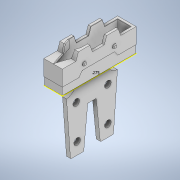
# Autodesk Inventor part: full bracket
Saved by Autodesk Inventor 2021 (Build 250183000, 183)
## iProperties
Created: 2021-07-17
Part Number: full bracket
Material: Generic
Document SubType Name: Modeling
Designer: newic
Density: 1 g/cm^3
Appearance: Default
Author: newic
Autodesk Inventor part; units mm, degrees
ref_plane "YZ Plane" through (0, 0, 0) normal (1, 0, 0) x (0, 1, 0)
ref_plane "XZ Plane" through (0, 0, 0) normal (0, 1, 0) x (-1, 0, 0)
sketch "Sketch1" plane through (0, 0, 0) normal (0, 1, 0) x (-1, 0, 0)
  line L0 (0, 0) -> (17.78, 0)
  line L1 (17.78, 0) -> (17.78, -71.12)
  line L2 (17.78, -71.12) -> (0, -71.12)
  line L3 (0, -71.12) -> (0, 0)
  dimension "d0" = 71.12
  dimension "d1" = 17.78
  constraints: 8 end point, 2 parallel, 1 horizontal, 1 perpendicular
  measures "d0" distance of L0.end L1.end
  measures "d1" distance of L1.end L2.end
extrude "Extrusion1" add sketch "Sketch1" along normal blind 31.75
sketch "Sketch2" plane through (0, 0, 0) normal (1, 0, 0) x (0, 0, -1)
  line L0 (63.2681, 31.9521) -> (6.1181, 31.9521)
  line L1 (2.3767, 22.4271) -> (69.8708, 22.4271)
  line L2 (34.6931, 31.9521) -> (34.6931, 22.4271)
  line L3 (3.5781, 31.9521) -> (3.5781, 0.2021)
  line L4 (3.5781, 22.4271) -> (11.8331, 22.4271)
  line L5 (65.8081, 31.9521) -> (65.8081, 0.2021)
  line L6 (65.8081, 22.4271) -> (57.5531, 22.4271)
  line L7 (34.6931, 22.4271) -> (38.5031, 22.4271)
  line L8 (34.6931, 22.4271) -> (30.8831, 22.4271)
  line L9 (3.5781, 22.4271) -> (13.1031, 22.4271)
  line L10 (34.6931, 22.4271) -> (28.9781, 22.4271)
  line L11 (34.6931, 22.4271) -> (40.4081, 22.4271)
  line L12 (65.8081, 22.4271) -> (56.2831, 22.4271)
  line L13 (3.5781, 37.1802) -> (21.3581, 37.1802)
  line L14 (21.3581, 37.1802) -> (21.3581, 22.4271)
  line L15 (21.3581, 31.9521) -> (21.3581, 29.4121)
  line L16 (3.5781, 29.4121) -> (65.8081, 29.4121)
  line L17 (40.4081, 22.4271) -> (47.996, 43.2748)
  line L18 (56.2831, 22.4271) -> (51.7026, 35.0119)
  line L19 (13.1031, 22.4271) -> (18.1209, 36.2135)
  line L20 (28.9781, 22.4271) -> (24.6631, 34.2823)
  line L21 (40.4081, 22.4271) -> (56.2831, 22.4271)
  line L22 (-0.2496, 29.1143) -> (71.3808, 29.1143)
  line L23 (71.3808, 29.1143) -> (71.3808, 39.1409)
  line L24 (71.3808, 39.1409) -> (-0.2496, 39.1409)
  line L25 (-0.2496, 39.1409) -> (-0.2496, 29.1143)
  line L26 (2.3767, 22.4271) -> (-0.2496, 29.1143)
  line L27 (68.8531, 22.4271) -> (71.3808, 29.1143)
  line L28 (2.3767, 22.4271) -> (-8.5713, 22.4271)
  line L29 (-8.5713, 22.4271) -> (69.8708, 22.4271)
  line L30 (76.0387, 22.4271) -> (71.3808, 31.956)
  line L31 (69.8708, 22.4271) -> (76.0387, 22.4271)
  line L32 (71.12, 0) -> (71.12, 31.75) projected
  line L33 (-7.4424, 22.4271) -> (-0.2496, 37.0193)
  point P0 (0, 0)
  point P1 (15.537, 29.1143)
  point P2 (26.5441, 29.1143)
  point P3 (42.842, 29.1143)
  point P4 (53.8491, 29.1143)
  dimension "d4" = 9.525
  dimension "d5" = 5.715
  dimension "d6" = 5.715
  dimension "d7" = 9.525
  dimension "d8" = 17.78
  dimension "d9" = 2.54
  dimension "d10" = 70
  dimension "d11" = 70
  dimension "d12" = 70
  dimension "d13" = 70
  constraints: 64 end point, 12 point on line, 5 horizontal, 3 perpendicular, 2 parallel, 2 vertical, 1 midpoint, 16 other
  measures "d4" distance of L4.start L19.start
  measures "d5" distance of L2.end L20.start
  measures "d6" distance of L2.end L17.start
  measures "d7" distance of L6.start L21.end
  measures "d8" distance of L13.start L14.start
  measures "d9" distance of L15.start L15.end
  measures "d10" angle to the sketch x axis of L19
  measures "d11" angle to the sketch x axis of L20
  measures "d12" angle to the sketch x axis of L17
  measures "d13" angle to the sketch x axis of L18
extrude "Extrusion2" cut sketch "Sketch2" against normal blind 31.75 contours L18 L16 L17 L0 | L0 L17 L24 L23 L22 L5 L16 L18 | L17 L16 L2 L0 | L0 L19 L16 L3 L22 L25 L24 L17 | L18 L22 L17 L16 | L16 L5 L22 L18 | L2 L16 L20 L0 | L17 L22 L2 L16 | L22 L5 L1 L18 | L20 L16 L14 L0 | L2 L22 L20 L16 | L17 L1 L2 L22 | L22 L32 L27 L1 L5 | L14 L16 L19 L0 | L20 L22 L14 L16 | L2 L1 L20 L22 | L25 L26 L28 L33 | L22 L27 L32 | L14 L22 L19 L16 | L22 L3 L1 L26 | L19 L22 L3 L16 | L22 L19 L1 L3
sketch "Sketch3" plane through (0, 0, 0) normal (1, 0, 0) x (0, 0, -1)
  line L0 (68.8531, 22.4271) -> (56.2831, 22.4271) projected
  line L1 (58.4871, 22.4271) -> (81.641, 22.4271)
  line L2 (81.641, 22.4271) -> (81.641, 34.8647)
  line L3 (81.641, 34.8647) -> (58.4871, 34.8647)
  line L4 (58.4871, 34.8647) -> (58.4871, 22.4271)
  point P0 (0, 0)
  constraints: 8 end point, 2 parallel, 1 horizontal, 1 perpendicular, 1 point on line
extrude "Extrusion3" cut sketch "Sketch3" against normal blind 31.75
sketch "Sketch4" plane through (0, 29.1143, -15.537) normal (0, 1, 0) x (1, 0, 0)
  line L0 (0, -15.537) -> (-17.78, -15.537) projected
  line L1 (0, -2.434) -> (0, -15.537) projected
  line L2 (0, -2.434) -> (-17.78, -2.434) projected
  line L3 (-17.78, -15.537) -> (-17.78, -2.434) projected
  line L4 (-17.78, 13.441) -> (-17.78, 24.871) projected
  line L5 (0, 13.441) -> (-17.78, 13.441) projected
  line L6 (0, 24.871) -> (0, 13.441) projected
  line L7 (0, 24.871) -> (-17.78, 24.871) projected
  line L8 (-17.78, 40.746) -> (-17.78, 55.583) projected
  line L9 (0, 40.746) -> (-17.78, 40.746) projected
  line L10 (0, 55.583) -> (0, 40.746) projected
  line L11 (-17.78, 55.583) -> (0, 55.583) projected
  line L12 (-15.24, -12.997) -> (-2.54, -12.997)
  line L13 (-2.54, -12.997) -> (-2.54, -4.974)
  line L14 (-2.54, -4.974) -> (-15.24, -4.974)
  line L15 (-15.24, -4.974) -> (-15.24, -12.997)
  line L16 (-15.24, -4.974) -> (-15.24, 52.7376)
  line L17 (-8.89, -12.997) -> (-15.24, 6.3053)
  line L18 (-8.89, -12.997) -> (-8.89, 3.3229)
  line L19 (-8.89, -12.997) -> (-2.54, 6.3053)
  line L20 (-2.54, 53.043) -> (-2.54, 43.286)
  line L21 (-2.54, 43.286) -> (-15.24, 43.286)
  line L22 (-15.24, 43.286) -> (-15.24, 53.043)
  line L23 (-15.24, 53.043) -> (-2.54, 53.043)
  line L24 (-2.54, -4.974) -> (-2.54, 53.043)
  point P0 (-2.54, 6.3053)
  point P1 (-15.24, 6.3053)
  dimension "d18" = 2.54
  dimension "d20" = 20.32
  dimension "d21" = 2.54
  constraints: 26 end point, 2 vertical, 1 midpoint, 1 symmetric about line, 6 other
  measures "d18" distance between parallel lines of L0 L12
  measures "d20" distance of L17.start L17.end
  measures "d21" distance between parallel lines of L11 L23
extrude "Extrusion4" cut sketch "Sketch4" against normal blind 26.67 contours L19 L14 L18 L2 | L2 L17 L16 L5 L24 L19 | L2 L18 L14 L17 | L19 L18 L14 | L5 L16 L7 L24 | L14 L18 L17 | L7 L16 L9 L24 | L9 L16 L21 L24 | L21 L16 L22 L23 L20
ref_plane "Work Plane1" through (0, 2.54, 0) normal (0, -1, 0) x (1, 0, 0)
sketch "Sketch5" plane through (0, 2.54, 0) normal (0, -1, 0) x (1, 0, 0)
  line L0 (-5.415, -13.1031) -> (-8.89, -2.54) projected
  line L1 (-8.89, -2.54) -> (-12.365, -13.1031) projected
  line L2 (-12.365, -13.1031) -> (-17.78, -13.1031) projected
  line L3 (-17.78, 0) -> (-17.78, -13.1031) projected
  line L4 (0, 0) -> (-17.78, 0) projected
  line L5 (0, -13.1031) -> (0, 0) projected
  line L6 (0, -13.1031) -> (-5.415, -13.1031) projected
  line L7 (-15.24, -2.54) -> (-15.24, -10.5631)
  line L8 (-15.24, -10.5631) -> (-14.2033, -10.5631)
  line L9 (-14.2033, -10.5631) -> (-8.89, 5.588)
  line L10 (-8.89, 5.588) -> (-3.5767, -10.5631)
  line L11 (-3.5767, -10.5631) -> (-2.54, -10.5631)
  line L12 (-2.54, -10.5631) -> (-2.54, -2.54)
  line L13 (-2.54, -2.54) -> (-15.24, -2.54)
  line L14 (-2.54, -68.58) -> (-2.54, -21.8423) projected
  line L15 (-15.24, -2.54) -> (-2.54, -2.54)
  line L16 (-2.54, -2.54) -> (-2.54, -68.58)
  line L17 (-2.54, -68.58) -> (-15.24, -68.58)
  line L18 (-15.24, -68.58) -> (-15.24, -2.54)
  point P0 (-2.54, -21.8423)
  dimension "d25" = 2.54
  constraints: 22 end point, 2 parallel, 1 horizontal, 1 perpendicular, 6 other
  measures "d25" distance between parallel lines of L4 L13
extrude "Extrusion5" cut sketch "Sketch5" against normal blind 17.78 contours L6 L16 L14 L17 L18 L2 L1 L0 | L0 L13 L10 L11 L16 L6 | L1 L2 L18 L8 L9 L13 | L13 L12 L11 L10 | L9 L8 L7 L13
sketch "Sketch6" plane through (0, 0, 0) normal (0, -1, 0) x (1, 0, 0)
  line L0 (0, -71.12) -> (-17.78, -71.12) projected
  line L1 (0, 0) -> (0, -71.12) projected
  line L2 (-17.78, 0) -> (0, 0) projected
  line L3 (-17.78, -71.12) -> (-17.78, 0) projected
  line L4 (-6.985, -64.135) -> (-10.795, -64.135)
  line L5 (-10.795, -64.135) -> (-10.795, -6.985)
  line L6 (-10.795, -6.985) -> (-6.985, -6.985)
  line L7 (-6.985, -6.985) -> (-6.985, -64.135)
  dimension "d28" = 6.985
  constraints: 8 end point, 3 other
  measures "d28" distance between parallel lines of L1 L7
sketch "Sketch7" plane through (0, 0, 0) normal (1, 0, 0) x (0, 0, -1)
  line L0 (4.699, 0) -> (66.421, 0)
  line L1 (4.699, 0) -> (4.699, -76.0491)
  line L2 (66.421, -76.0491) -> (4.699, -76.0491)
  line L3 (66.421, 0) -> (66.421, -76.0491)
  line L4 (4.699, 0) -> (66.421, 0)
  line L5 (4.699, 0) -> (11.049, 0)
  line L6 (11.049, 0) -> (11.049, -11.43)
  line L7 (4.445, 0) -> (57.277, 0)
  line L8 (66.421, 0) -> (60.071, 0)
  line L9 (60.071, 0) -> (60.071, -11.43)
  line L10 (4.699, 0) -> (4.699, -63.5)
  line L11 (4.699, 0) -> (4.699, -76.0491)
  line L12 (66.421, 0) -> (66.421, -76.0491)
  line L13 (14.859, -63.5) -> (26.9853, -63.5)
  line L14 (55.6708, -63.5) -> (43.561, -63.5)
  line L15 (11.049, -11.43) -> (14.8159, -62.9113)
  line L16 (27.617, -62.9292) -> (31.3898, -25.8199)
  line L17 (32.0216, -25.2491) -> (39.0985, -25.2491)
  line L18 (39.7302, -25.8199) -> (43.503, -62.9292)
  line L19 (56.3041, -62.9113) -> (60.071, -11.43)
  line L20 (11.049, 0) -> (21.209, 0)
  line L21 (60.071, 0) -> (49.911, 0)
  arc A0 (11.049, -11.43) -> (21.209, 0) centre (9.7792, -0.0708) ccw
  arc A1 (49.911, 0) -> (60.071, -11.43) centre (61.3408, -0.0708) ccw
  arc A2 (32.0216, -25.2491) -> (31.3898, -25.8199) centre (32.0216, -25.8841) ccw
  arc A3 (39.7302, -25.8199) -> (39.0985, -25.2491) centre (39.0985, -25.8841) ccw
  arc A4 (26.9853, -63.5) -> (27.617, -62.9292) centre (26.9853, -62.865) ccw
  arc A5 (14.8159, -62.9113) -> (15.4492, -63.5) centre (15.4492, -62.865) ccw
  arc A6 (43.503, -62.9292) -> (44.1347, -63.5) centre (44.1347, -62.865) ccw
  arc A7 (55.6708, -63.5) -> (56.3041, -62.9113) centre (55.6708, -62.865) ccw
  line L22 (51.1504, -63.5) -> (51.1504, -52.07)
  circle A8 centre (20.32, -19.05) radius 3.175
  circle A9 centre (50.8, -19.05) radius 3.175
  circle A10 centre (21.209, -52.07) radius 3.175
  line L23 (71.12, 0) -> (0, 0) projected
  line L24 (66.421, 0) -> (71.12, 0)
  line L25 (71.12, 0) -> (66.421, 0)
  line L26 (66.421, 0) -> (66.421, 0.7466)
  line L27 (35.56, -25.2491) -> (35.56, 0)
  line L28 (26.5441, 29.1143) -> (15.537, 29.1143) projected
  line L29 (50.8, -63.5) -> (50.8, -52.07)
  circle A11 centre (50.8, -52.07) radius 3.175
  point P0 (27.559, -63.5)
  point P1 (50.8, -55.245)
  point P2 (51.1504, -55.2256)
  point P3 (15.4492, -63.5)
  dimension "d0" = 71.12
  dimension "d1" = 17.78
  dimension "d4" = 9.525
  dimension "d29" = 6.35
  dimension "d30" = 11.43
  dimension "d31" = 6.35
  dimension "d32" = 11.43
  dimension "d33" = 63.5
  dimension "d34" = 10.16
  dimension "d36" = 12.7
  dimension "d41" = 10.16
  dimension "d42" = 10.16
  dimension "d43" = 11.43
  dimension "d44" = 11.43
  dimension "d45" = 0.635
  dimension "d47" = 11.43
  dimension "d52" = 6.35
  dimension "d53" = 6.35
  dimension "d55" = 4.699
  dimension "d56" = 180
  dimension "d57" = 90
  dimension "d58" = 15.24
  dimension "d59" = 15.24
  dimension "d60" = 11.43
  dimension "d61" = 6.35
  constraints: 56 end point, 16 point on circle, 12 centre point, 11 point on line, 10 tangent, 5 equal radius, 3 perpendicular, 2 horizontal, 1 coincident, 1 midpoint, 1 vertical, 2 other
  measures "d29" distance of L10.start L5.end
  measures "d30" distance of L5.end L15.start
  measures "d31" distance of L3.start L9.start
  measures "d32" distance of L9.start L19.end
  measures "d33" distance of L10.start L10.end
  measures "d34" distance of L10.end L13.start
  measures "d36" distance of L13.start point (27.559, -63.5)
  measures "d41" distance of L5.end L20.end
  measures "d42" distance of L9.start L21.end
  measures "d43" radius of A0
  measures "d44" radius of A1
  measures "d45" radius of A2
  measures "d47" distance of L22.start L22.end
  measures "d52" diameter of A9
  measures "d53" diameter of A10
  measures "d55" distance of L24.end L25.end
  measures "d56" angle of L3 L27
  measures "d57" angle of L28 L27
  measures "d58" distance from line of A8.centre L27
  measures "d59" distance from line of A9.centre L27
  measures "d60" distance of L29.start L29.end
  measures "d61" diameter of A11
extrude "Extrusion6" add sketch "Sketch7" against normal blind 17.78 contours L0 L27 L17 A2 L16 A4 L13 A5 L15 A0 | L0 A1 L19 A7 L14 L22 A11 L29 A6 L18 A3 L17 L27
sketch "Sketch8" plane through (0, 0, -71.12) normal (0, 0, -1) x (-1, 0, 0)
  line L0 (17.78, 0) -> (0, 0) projected
  line L1 (8.89, 0) -> (8.89, -149.5828)
  line L2 (10.795, 0) -> (10.795, -149.5828)
  line L3 (6.985, 0) -> (6.985, -149.5828)
  line L4 (6.985, -79.5842) -> (-31.3373, 0)
  line L5 (-31.3373, 0) -> (44.0214, 0)
  line L6 (44.0214, 0) -> (10.795, -80.7526)
  dimension "d64" = 1.905
  dimension "d65" = 1.905
  constraints: 12 end point, 2 parallel, 2 point on line, 1 horizontal, 1 midpoint, 1 vertical
  measures "d64" distance between parallel lines of L1 L2
  measures "d65" distance between parallel lines of L1 L3
extrude "Extrusion7" cut sketch "Sketch8" against normal blind 508
sketch "Sketch9" plane through (-6.985, -63.5, -51.1504) normal (1, 0, 0) x (0, 0, -1)
  arc A0 (0, 8.2744) -> (-0.3504, 8.255) centre (-0.3504, 11.43) ccw projected
  circle A1 centre (-0.3504, 11.43) radius 3.175
  line L0 (-7.0156, 0) -> (-0.3504, 0) projected
  line L1 (-0.6355, 0) -> (0.8386, 0)
  line L2 (-0.4861, 0) -> (-1.3257, 8.4085)
  line L3 (0, 0) -> (4.5204, 0) projected
  line L4 (0.4648, 0) -> (0.4648, 8.3614)
  point P0 (-51.1504, 63.5)
  point P1 (0.4648, 0)
  point P2 (0.4648, 8.3614)
  point P3 (-0.3504, 8.255)
  point P4 (-1.3257, 8.4085)
  point P5 (-0.4861, 0)
  constraints: 6 end point, 3 point on line, 2 point on circle, 1 centre point, 1 coincident, 1 collinear, 1 perpendicular
extrude "Extrusion8" add sketch "Sketch9" against normal blind 3.81 contours A0 L4 L1 L0 L2 A1
sketch "Sketch10" plane through (0, 0, 0) normal (1, 0, 0) x (0, 0, -1)
  line L0 (3.653, 22.2211) -> (3.653, -0.0039)
  line L1 (3.653, 22.2211) -> (3.653, -0.0039)
  line L2 (3.653, -0.0039) -> (3.653, 7.3621)
  line L3 (3.653, 7.3621) -> (65.883, 7.3621)
  line L4 (65.883, 22.2211) -> (65.883, -0.0039)
  line L5 (15.687, 29.1143) -> (26.5441, 29.1143)
  line L6 (21.1155, 29.1143) -> (21.1155, 4.5403)
  line L7 (53.8491, 29.1143) -> (42.992, 29.1143)
  line L8 (48.4205, 29.1143) -> (48.4205, 5.1354)
  line L9 (21.1155, 7.3621) -> (17.9405, 7.3621)
  line L10 (48.4205, 7.3621) -> (51.5955, 7.3621)
  line L11 (51.5955, 7.3621) -> (51.5955, 11.8071)
  line L12 (17.9405, 7.3621) -> (17.9405, 11.8071)
  line L13 (21.1155, 11.8071) -> (48.4205, 11.8071)
  line L14 (3.653, 7.3621) -> (3.653, 22.2211)
  line L15 (3.653, 14.7916) -> (68.0217, 14.7916)
  line L16 (3.653, 16.6966) -> (68.0217, 16.6966)
  circle A0 centre (21.1155, 16.6966) radius 1.905
  circle A1 centre (48.4205, 16.6966) radius 1.905
  line L17 (50.3255, 11.8071) -> (53.5005, 7.3621)
  line L18 (19.2105, 11.8071) -> (16.0355, 7.3621)
  line L19 (19.2105, 11.8071) -> (21.1155, 11.8071)
  line L20 (50.3255, 11.8071) -> (48.4205, 11.8071)
  line L21 (16.5523, 6.9931) -> (19.5373, 11.1721)
  line L22 (19.5373, 11.1721) -> (21.1155, 11.1721)
  line L23 (21.1155, 11.1721) -> (48.4205, 11.1721)
  line L24 (48.4205, 11.1721) -> (49.9988, 11.1721)
  line L25 (49.9988, 11.1721) -> (52.9838, 6.9931)
  line L26 (3.653, 6.7271) -> (65.883, 6.7271)
  line L27 (16.5523, 6.9931) -> (16.3623, 6.7271)
  line L28 (52.9838, 6.9931) -> (53.5005, 6.3456)
  line L29 (3.653, 7.3621) -> (-3.2474, 7.3621)
  line L30 (3.653, 6.7271) -> (-3.0258, 6.7271)
  line L31 (65.883, 7.3621) -> (72.9807, 7.3621)
  line L32 (65.883, 6.7271) -> (72.9807, 6.7271)
  line L33 (72.9807, 7.3621) -> (72.9807, -12.768)
  line L34 (72.9807, -12.768) -> (-11.8016, -10.0683)
  line L35 (-11.8016, -10.0683) -> (-3.2474, 7.3621)
  point P0 (0, 0)
  point P1 (6.193, 31.7461)
  dimension "d70" = 7.366
  dimension "d71" = 3.175
  dimension "d72" = 3.175
  dimension "d73" = 4.445
  dimension "d74" = 4.445
  dimension "d75" = 1.905
  dimension "d76" = 0.635
  dimension "d77" = 0.635
  constraints: 72 end point, 17 point on line, 4 perpendicular, 4 vertical, 3 horizontal, 3 midpoint, 2 centre point, 2 collinear, 2 parallel, 4 other
  measures "d70" distance of L0.end L3.start
  measures "d71" distance of L9.start L9.end
  measures "d72" distance of L10.start L10.end
  measures "d73" distance of L10.end L11.end
  measures "d74" distance of L9.end L12.end
  measures "d75" distance between parallel lines of L15 L16
  measures "d76" distance between parallel lines of L18 L21
  measures "d77" distance between parallel lines of L3 L26
extrude "Extrusion9" cut sketch "Sketch10" against normal blind 0.3175 contours L3 L21 L27 L26 L0 | L0 L26 L32 L33 L34 L35 L29 | L18 L12 L21 L3 | L13 L8 L23 L6 | L6 L22 L21 L12 L18 L19 | L27 L21 L3 L6 L26 | L21 L12 L3 | L23 L8 L3 L6 | L6 L3 L12 L21 L22 | L20 L17 L11 L25 L24 L8 | L6 L3 L8 L26 | L24 L25 L11 L3 L8 | L4 L26 L28 L25 L3 | L31 L33 L32 L4 | L8 L3 L25 L28 L26 | L17 L3 L25 L11 | L11 L25 L3
sketch "Sketch11" plane through (-17.78, 0, -71.12) normal (-1, 0, 0) x (0, 0, 1)
  line L0 (51.9095, 11.8071) -> (20.7945, 11.8071) projected
  line L1 (20.7945, 11.8071) -> (17.6195, 7.3621) projected
  line L2 (17.6195, 7.3621) -> (0, 7.3621) projected
  line L3 (55.0845, 7.3621) -> (51.9095, 11.8071) projected
  line L4 (71.12, 7.3621) -> (55.0845, 7.3621) projected
  line L5 (0, 0) -> (0, 22.4271) projected
  line L6 (71.12, 0) -> (71.12, 22.4271) projected
  line L7 (0, 7.3621) -> (0, 0) projected
  line L8 (0, 0) -> (71.12, 0)
  line L9 (71.12, 0) -> (71.12, 7.3621)
  line L10 (71.12, 7.3621) -> (0, 7.3621)
  line L11 (0, 7.3621) -> (0, 0)
  line L12 (20.7945, 11.8071) -> (51.9095, 11.8071)
  line L13 (55.0845, 7.3621) -> (51.9095, 11.8071) projected
  line L14 (55.0845, 7.3621) -> (51.9095, 11.8071)
  line L15 (20.7945, 11.8071) -> (17.6195, 7.3621)
  constraints: 14 end point, 4 equal length, 1 horizontal, 1 perpendicular, 1 point on line
extrude "Extrusion10" cut sketch "Sketch11" against normal blind 0.3175
sketch "Sketch12" plane through (0, 22.4271, -71.12) normal (0, 0, -1) x (-1, 0, 0)
  line L0 (17.78, -15.0649) -> (17.4625, -15.0649) projected
  line L1 (0, -22.4271) -> (17.78, -22.4271)
  line L2 (17.78, -22.4271) -> (17.78, -15.0649)
  line L3 (17.78, -15.0649) -> (0, -15.0649)
  line L4 (0, -15.0649) -> (0, -22.4271)
  constraints: 8 end point, 2 parallel, 1 horizontal, 1 perpendicular
extrude "Extrusion11" cut sketch "Sketch12" against normal blind 0.3175
sketch "Sketch13" plane through (-17.78, 22.4271, 0) normal (0, 0, 1) x (1, 0, 0)
  line L0 (0, -15.0649) -> (0.3175, -15.0649) projected
  line L1 (0.3175, -15.0649) -> (0.3175, -22.4271) projected
  line L2 (0.3175, -22.4271) -> (17.4625, -22.4271) projected
  line L3 (17.4625, -22.4271) -> (17.4625, -15.0649) projected
  line L4 (17.4625, -15.0649) -> (17.78, -15.0649) projected
  line L5 (17.78, -15.0649) -> (17.78, 0) projected
  line L6 (17.78, 0) -> (0, 0) projected
  line L7 (0, -15.0649) -> (0, 0) projected
  line L8 (0.3175, -22.4271) -> (17.4625, -22.4271) projected
  line L9 (17.78, -15.0649) -> (17.78, 0) projected
  line L10 (0.3175, -22.4271) -> (17.78, -22.4271)
  line L11 (17.78, -22.4271) -> (17.78, -15.0649)
  line L12 (17.78, -15.0649) -> (0.3175, -15.0649)
  line L13 (0.3175, -15.0649) -> (0.3175, -22.4271)
  constraints: 8 end point, 2 parallel, 1 horizontal, 1 perpendicular
extrude "Extrusion12" cut sketch "Sketch13" against normal blind 0.3175 contours L12 L3 L2 L1
sketch "Sketch14" plane through (0, 22.4271, -56.2831) normal (1, 0, 0) x (0, 0, -1)
  line L0 (-34.4407, 6.6873) -> (-29.739, 6.6873) projected
  line L1 (-34.4407, 6.6873) -> (-34.4407, -5.7587)
  line L2 (-34.4407, 6.6873) -> (-34.4407, -2.1071) projected
  line L3 (-2.434, 6.6873) -> (-13.441, 6.6873) projected
  line L4 (-8.9424, 6.6873) -> (-8.9424, -5.7587)
  line L5 (-56.2831, -15.0649) -> (-56.2831, 0) projected
  line L6 (-56.2831, -5.7587) -> (-35.2011, -5.7587)
  line L7 (14.8369, -5.7587) -> (14.8369, -26.8407)
  line L8 (14.8369, -5.7587) -> (-6.2451, -5.7587)
  circle A0 centre (-35.2011, -5.7587) radius 1.905
  circle A1 centre (-6.2451, -5.7587) radius 1.905
  point P0 (-56.2831, -22.4271)
  dimension "d94" = 12.446
  dimension "d96" = 12.446
  dimension "d97" = 21.082
  dimension "d98" = 21.082
  dimension "d99" = 21.082
  dimension "d100" = 3.81
  dimension "d101" = 3.81
  constraints: 10 end point, 2 centre point, 2 coincident, 2 perpendicular, 2 point on line, 1 collinear, 1 horizontal
  measures "d94" distance of L0.start L1.end
  measures "d96" distance of L4.start L4.end
  measures "d97" distance of L6.start L6.end
  measures "d98" distance of L7.start L7.end
  measures "d99" distance of L7.start L8.end
  measures "d100" diameter of A0
  measures "d101" diameter of A1
extrude "Extrusion13" add sketch "Sketch14" along normal blind 1.27 and the other way blind 19.05
sketch "Sketch15" plane through (0, 2.4443, -15.537) normal (0, 1, 0) x (1, 0, 0)
  line L0 (-2.54, 53.043) -> (-2.54, 6.3053) projected
  line L1 (-15.24, 6.3053) -> (-15.24, -12.997) projected
  line L2 (-2.54, 45.996) -> (-15.24, 45.996)
  line L3 (-15.24, 45.996) -> (-15.24, 0.868)
  line L4 (-15.24, 0.868) -> (-2.54, 0.868)
  line L5 (-2.54, 0.868) -> (-2.54, 45.996)
  point P0 (0, -15.537)
  point P1 (-2.54, 6.3053)
  constraints: 8 end point, 2 parallel, 2 point on line, 1 horizontal, 1 perpendicular
extrude "Extrusion14" cut sketch "Sketch15" along normal blind 16.51
fillet "Fillet1" radius 0.762 2 edges at (1.27, 16.6683, -48.133) (1.27, 16.6683, -19.177)
fillet "Fillet2" radius 0.762 2 edges at (-19.05, 16.6683, -48.133) (-19.05, 16.6683, -19.177)
fillet "Fillet3" radius 0.762 8 edges at (-3.5771, 29.1143, -18.6897) (-5.0146, 25.7707, -14.3201) (-7.1525, 22.4271, -7.8215) (-10.6275, 22.4271, -7.8215) (-12.7654, 25.7707, -14.3201) (-14.2029, 29.1143, -18.6897) (-12.065, 20.32, -12.1912) (-5.715, 20.32, -12.1912)
fillet "Fillet4" radius 0.254 15 edges at (-15.24, 22.4271, -34.6931) (-2.54, 22.4271, -34.6931) (-2.54, 25.7707, -27.7611) (-2.54, 29.1143, -22.974) (-2.54, 25.7707, -41.6251) (-2.54, 29.1143, -48.3456) (-2.54, 25.7707, -55.0661) (-2.54, 22.4271, -62.4315) (-8.89, 22.4271, -68.58) (-15.24, 22.4271, -62.4315) (-15.24, 25.7707, -55.0661) (-15.24, 29.1143, -48.3456) (-15.24, 25.7707, -41.6251) (-15.24, 25.7707, -27.7611) (-15.24, 29.1143, -22.974)
body "Solid1"
